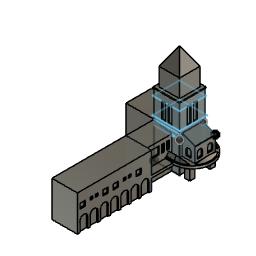
theater (Autodesk Fusion 360 design; units mm, degrees)
Autodesk Fusion 360 part; units mm, degrees
note: some values were not read from the file. Set by a fixed rule: which sketch regions a step uses.
sketch "Sketch1" plane through (0, 0, 0) normal (0, 0, 1) x (1, 0, 0)
  line L0 (-50, 50) -> (50, 50)
  line L1 (50, 50) -> (50, -50)
  line L2 (50, -50) -> (-50, -50)
  line L3 (-50, -50) -> (-50, 50)
  constraint horizontal L0
  constraint vertical L1
  constraint horizontal L2
  constraint vertical L3
extrude "Extrude1" add sketch "Sketch1" along normal blind 325
sketch "Sketch2" plane through (0, 0, 325) normal (0, 0, 1) x (-1, 0, 0)
  line L0 (50, 50) -> (-50, 50)
  line L1 (-50, 50) -> (-50, -50)
  line L2 (-50, -50) -> (50, -50)
  line L3 (50, -50) -> (50, 50)
  line L4 (40, -40) -> (-40, -40)
  line L5 (-40, -40) -> (-40, 40)
  line L6 (-40, 40) -> (40, 40)
  line L7 (40, 40) -> (40, -40)
  constraint horizontal L4
  constraint vertical L5
  constraint horizontal L6
  constraint vertical L7
extrude "Extrude2" cut sketch "Sketch2" against normal blind 50 contours L0 L1 L2 L3 | L4 L5 L6 L7
sketch "Sketch3" plane through (0, 0, 275) normal (0, 0, 1) x (-1, 0, 0)
  line L0 (50, -50) -> (50, 50)
  line L1 (50, 50) -> (-50, 50)
  line L2 (-50, 50) -> (-50, -50)
  line L3 (-50, -50) -> (50, -50)
  line L4 (40, -40) -> (-40, -40)
  line L5 (-40, -40) -> (-40, 40)
  line L6 (-40, 40) -> (40, 40)
  line L7 (40, 40) -> (40, -40)
  constraint horizontal L4
  constraint vertical L5
  constraint horizontal L6
  constraint vertical L7
extrude "Extrude3" add sketch "Sketch3" along normal blind 70 contours L4 L5 L6 L7
extrude "Extrude4" cut 1 faces at (-13.3333, 13.3333, 345) along direction (0, 0, -1) blind 25
extrude "Extrude5" cut 1 faces at (46.6667, 13.3333, 275) along direction (0, 0, -1) blind 25
extrude "Extrude6" add 1 faces at (-13.3333, 13.3333, 320) along direction (0, 0, 1) blind 80 draft -30
sketch "Sketch4" plane through (0, 0, 0) normal (0, 0, 1) x (1, 0, 0)
sketch "Sketch5" plane through (0, 0, 250) normal (0, 0, 1) x (-1, 0, 0)
  line L0 (40, 40) -> (40, -40)
  line L1 (40, -40) -> (-40, -40)
  line L2 (-40, -40) -> (-40, 40)
  line L3 (-40, 40) -> (40, 40)
  line L4 (50, -50) -> (50, 50)
  line L5 (50, 50) -> (-50, 50)
  line L6 (-50, 50) -> (-50, -50)
  line L7 (-50, -50) -> (50, -50)
  line L8 (52, -52) -> (-52, -52)
  line L9 (-52, -52) -> (-52, 52)
  line L10 (-52, 52) -> (52, 52)
  line L11 (52, 52) -> (52, -52)
  constraint horizontal L8
  constraint vertical L9
  constraint horizontal L10
  constraint vertical L11
extrude "Extrude7" add sketch "Sketch5" against normal blind 3.5 contours L8 L9 L10 L11
extrude "Extrude8" add 1 faces at (-16.6667, 51.3333, 246.5) along direction (0, 0, -1) blind 5 draft -60
sketch "Sketch6" plane through (50, 0, 0) normal (1, 0, 0) x (0, 1, 0)
  line L0 (50, 246.5) -> (-50, 246.5)
  line L1 (-50, 246.5) -> (-50, 0)
  line L2 (-50, 0) -> (50, 0)
  line L3 (50, 0) -> (50, 246.5)
  line L4 (-40, 120) -> (40, 120)
  line L5 (40, 120) -> (40, 60)
  line L6 (40, 60) -> (-40, 60)
  line L7 (-40, 60) -> (-40, 120)
  line L8 (-40, 100) -> (40, 100)
  line L9 (40, 100) -> (40, 60)
  line L10 (40, 60) -> (-40, 60)
  line L11 (-40, 60) -> (-40, 100)
  constraint horizontal L4
  constraint vertical L5
  constraint horizontal L6
  constraint vertical L7
  constraint horizontal L8
  constraint vertical L9
  constraint horizontal L10
  constraint vertical L11
  constraint coincident L7 L8.start
extrude "Extrude9" add sketch "Sketch6" along normal blind 50 contours L4 L5 L7 L8 | L5 L6 L7 L8 L9 L10 L11
sketch "Sketch7" plane through (100, 0, 0) normal (1, 0, 0) x (0, 1, 0)
  line L0 (-40, 60) -> (40, 60)
  line L1 (40, 60) -> (40, 120)
  line L2 (40, 120) -> (-40, 120)
  line L3 (-40, 120) -> (-40, 60)
  line L4 (-40, 120) -> (40, 120)
  line L5 (40, 120) -> (40, 100)
  line L6 (40, 100) -> (-40, 100)
  line L7 (-40, 100) -> (-40, 120)
  constraint horizontal L4
  constraint vertical L5
  constraint horizontal L6
  constraint vertical L7
  constraint coincident L1 L5.end
  constraint coincident L2.end L3.start
extrude "Extrude10" add sketch "Sketch7" against normal blind 50 draft 20 contours L1 L2 L3 L4 L5 L6 L7
sketch "Sketch8" plane through (50, 0, 0) normal (1, 0, 0) x (0, 1, 0)
  line L0 (-50, 138.1985) -> (50, 138.1985)
  line L1 (50, 138.1985) -> (50, 246.5)
  line L2 (50, 246.5) -> (-50, 246.5)
  line L3 (-50, 246.5) -> (-50, 138.1985)
  line L4 (-40, 60) -> (-60, 60)
  line L5 (-60, 60) -> (-60, 140)
  line L6 (-60, 140) -> (-40, 140)
  line L7 (-40, 140) -> (-40, 60)
  line L8 (60, 60) -> (40, 60)
  line L9 (40, 60) -> (40, 140)
  line L10 (40, 140) -> (60, 140)
  line L11 (60, 140) -> (60, 60)
  constraint horizontal L4
  constraint vertical L5
  constraint horizontal L6
  constraint vertical L7
  constraint horizontal L8
  constraint vertical L9
  constraint horizontal L10
  constraint vertical L11
extrude "Extrude11" cut sketch "Sketch8" along normal blind 140 contours L0 L1 L8 L9 L10 L11
sketch "Sketch9" plane through (50, 0, 0) normal (1, 0, 0) x (0, 1, 0)
  line L0 (-50, 138.1985) -> (40, 138.1985)
  line L1 (40, 138.1985) -> (40, 60)
  line L2 (40, 60) -> (-40, 60)
  line L3 (-40, 60) -> (-40, 81.8015)
  line L4 (-40, 81.8015) -> (-50, 81.8015)
  line L5 (-50, 81.8015) -> (-50, 0)
  line L6 (-50, 0) -> (50, 0)
  line L7 (50, 0) -> (50, 246.5)
  line L8 (50, 246.5) -> (-50, 246.5)
  line L9 (-50, 246.5) -> (-50, 138.1985)
  line L10 (-40, 60) -> (-61.5623, 60)
  line L11 (-61.5623, 60) -> (-61.5623, 138.1985)
  line L12 (-61.5623, 138.1985) -> (-40, 138.1985)
  line L13 (-40, 138.1985) -> (-40, 60)
  constraint horizontal L10
  constraint vertical L11
  constraint horizontal L12
  constraint vertical L13
  constraint coincident L2.end L3.start
extrude "Extrude12" cut sketch "Sketch9" along normal blind 320 contours L0 L4 L5 L10 L11 L12 L13
sketch "Sketch10" plane through (100, 0, 0) normal (1, 0, 0) x (0, 1, 0)
  line L0 (-40, 120) -> (-40, 60)
  line L1 (-40, 60) -> (40, 60)
  line L2 (40, 60) -> (40, 120)
  line L3 (40, 120) -> (-40, 120)
  line L4 (-30, 70) -> (-10, 70)
  line L5 (-10, 70) -> (-10, 90)
  line L6 (-10, 90) -> (-30, 90)
  line L7 (-30, 90) -> (-30, 70)
  circle A0 centre (-20, 90) radius 10
  line L8 (-30, 90) -> (-10, 90)
  line L9 (-30, 90) -> (-10, 90)
  constraint horizontal L4
  constraint vertical L5
  constraint horizontal L6
  constraint vertical L7
  constraint midpoint L6 A0.centre
  constraint coincident L5.end A0
extrude "Extrude13" cut sketch "Sketch10" against normal blind 5 contours L4 L5 L7 A0 | L6 A0 L8 L9 | L6 A0 L8 L9
sketch "Sketch11" plane through (100, 0, 0) normal (1, 0, 0) x (0, 1, 0)
  line L0 (-30, 70) -> (-30, 90)
  arc A0 (-10, 90) -> (-30, 90) centre (-20, 90) ccw
  line L1 (-10, 90) -> (-10, 70)
  line L2 (-10, 70) -> (-30, 70)
  line L3 (-40, 120) -> (-40, 60)
  line L4 (-40, 60) -> (40, 60)
  line L5 (40, 60) -> (40, 120)
  line L6 (40, 120) -> (-40, 120)
  line L7 (10, 70) -> (30, 70)
  line L8 (30, 70) -> (30, 90)
  line L9 (30, 90) -> (10, 90)
  line L10 (10, 90) -> (10, 70)
  circle A1 centre (20, 90) radius 10
  constraint horizontal L7
  constraint vertical L8
  constraint horizontal L9
  constraint vertical L10
  constraint midpoint L9 A1.centre
  constraint coincident L8.end A1
extrude "Extrude14" cut sketch "Sketch11" against normal blind 5 contours L7 L8 L10 A1 | L9 A1 | L9 A1
sketch "Sketch12" plane through (0, 40, 0) normal (0, 1, 0) x (-1, 0, 0)
  line L0 (-100, 120) -> (-100, 60)
  line L1 (-100, 60) -> (-50, 60)
  line L2 (-50, 60) -> (-50, 138.1985)
  line L3 (-50, 138.1985) -> (-100, 120)
  line L4 (-85, 70) -> (-65, 70)
  line L5 (-65, 70) -> (-65, 90)
  line L6 (-65, 90) -> (-85, 90)
  line L7 (-85, 90) -> (-85, 70)
  circle A0 centre (-75, 90) radius 10
  constraint horizontal L4
  constraint vertical L5
  constraint horizontal L6
  constraint vertical L7
  constraint midpoint L6 A0.centre
  constraint coincident L5.end A0
extrude "Extrude15" cut sketch "Sketch12" against normal blind 5 contours L4 L5 L7 A0 | L6 A0 | L6 A0
sketch "Sketch13" plane through (0, -40, 0) normal (0, -1, 0) x (1, 0, 0)
  line L0 (50, 138.1985) -> (50, 60)
  line L1 (50, 60) -> (100, 60)
  line L2 (100, 60) -> (100, 120)
  line L3 (100, 120) -> (50, 138.1985)
sketch "Sketch14" plane through (0, -40, 0) normal (0, -1, 0) x (1, 0, 0)
  line L0 (65, 70) -> (85, 70)
  line L1 (85, 70) -> (85, 90)
  line L2 (85, 90) -> (65, 90)
  line L3 (65, 90) -> (65, 70)
  circle A0 centre (75, 90) radius 10
  constraint horizontal L0
  constraint vertical L1
  constraint horizontal L2
  constraint vertical L3
  constraint midpoint L2 A0.centre
  constraint coincident L1.end A0
extrude "Extrude16" cut sketch "Sketch14" against normal blind 5
sketch "Sketch15" plane through (50.265, 0, 138.102) normal (0.34202, 0, 0.939693) x (0, 1, 0)
  line L0 (-40, 0.282) -> (-40, -52.9268)
  line L1 (-40, -52.9268) -> (40, -52.9268)
  line L2 (40, -52.9268) -> (40, 0.282)
  line L3 (40, 0.282) -> (-40, 0.282)
sketch "Sketch16" plane through (100, 0, 0) normal (1, 0, 0) x (0, 1, 0)
  line L0 (10, 70) -> (10, 90)
  arc A0 (30, 90) -> (10, 90) centre (20, 90) ccw
  line L1 (30, 90) -> (30, 70)
  line L2 (30, 70) -> (10, 70)
  line L3 (-30, 70) -> (-30, 90)
  arc A1 (-10, 90) -> (-30, 90) centre (-20, 90) ccw
  line L4 (-10, 90) -> (-10, 70)
  line L5 (-10, 70) -> (-30, 70)
  line L6 (-40, 120) -> (-40, 60)
  line L7 (-40, 60) -> (40, 60)
  line L8 (40, 60) -> (40, 120)
  line L9 (40, 120) -> (-40, 120)
  line L10 (-40, 120) -> (40, 120)
  line L11 (40, 120) -> (40, 117.9644)
  line L12 (40, 117.9644) -> (-40, 117.9644)
  line L13 (-40, 117.9644) -> (-40, 120)
  constraint horizontal L10
  constraint vertical L11
  constraint horizontal L12
  constraint vertical L13
  constraint coincident L8 L11.end
  constraint coincident L6.start L9.end
extrude "Extrude17" add sketch "Sketch16" along normal blind 4 draft -20 contours L6 L8 L9 L10 L11 L12 L13
sketch "Sketch17" plane through (0, 40, 0) normal (0, 1, 0) x (-1, 0, 0)
  line L0 (-85, 70) -> (-85, 90)
  arc A0 (-65, 90) -> (-85, 90) centre (-75, 90) ccw
  line L1 (-65, 90) -> (-65, 70)
  line L2 (-65, 70) -> (-85, 70)
  line L3 (-100, 117.9644) -> (-100, 60)
  line L4 (-100, 60) -> (-50, 60)
  line L5 (-50, 60) -> (-50, 138.1985)
  line L6 (-50, 138.1985) -> (-100, 120)
  line L7 (-100, 120) -> (-100, 117.9644)
  line L8 (-100, 117.9644) -> (-50, 136.0984)
  constraint coincident L3.start L7.end
  constraint coincident L5 L8.end
ref_plane "WorkPlane1" through (0, 0, 60) normal (0, 0, 1) x (1, 0, 0)
sketch "Sketch18" plane through (0, 0, 60) normal (0, 0, 1) x (1, 0, 0)
  circle A0 centre (50, 0) radius 76.0694
extrude "Extrude18" add sketch "Sketch18" against normal blind 10
sketch "Sketch19" plane through (0, 0, 60) normal (0, 0, 1) x (-1, 0, 0)
  line L0 (-50, 50) -> (7.3284, 50)
  arc A0 (7.3284, 50) -> (7.3284, -50) centre (-50, 0) ccw
  line L1 (7.3284, -50) -> (-50, -50)
  line L2 (-50, -50) -> (-50, -40)
  line L3 (-50, -40) -> (-100, -40)
  line L4 (-100, -40) -> (-100, 40)
  line L5 (-100, 40) -> (-50, 40)
  line L6 (-50, 40) -> (-50, 50)
  line L7 (-104.9015, -44.9015) -> (-104.9015, 44.9015)
  line L8 (-54.9015, 54.9015) -> (-4.7156, 54.9015)
  arc A1 (-4.7156, 54.9015) -> (-4.7156, -54.9015) centre (-50, 0) ccw
  line L9 (-4.7156, -54.9015) -> (-54.9015, -54.9015)
  line L10 (-54.9015, 54.9015) -> (-95.2844, 54.9015)
  line L11 (-54.9015, -54.9015) -> (-95.2844, -54.9015)
  line L12 (-104.9015, 49.6433) -> (-104.9015, -50)
  constraint coincident A1 L10.end
  constraint concentric A0 A1
  constraint coincident A1 L11.end
  constraint parallel L7 L12
extrude "Extrude19" add sketch "Sketch19" along normal blind 20 draft -30 contours L7 A1 L12 | L8 A1 L10 | A1 L9 L11
sketch "Sketch20" plane through (0, 0, 50) normal (0, 0, -1) x (1, 0, 0)
  line L0 (-7.3284, 50) -> (50, 50)
  line L1 (50, 50) -> (50, -50)
  line L2 (50, -50) -> (-7.3284, -50)
  arc A0 (-7.3284, -50) -> (-7.3284, 50) centre (50, 0) ccw
  line L3 (90, 50) -> (70, 50)
  line L4 (70, 50) -> (70, 30)
  line L5 (70, 30) -> (90, 30)
  line L6 (90, 30) -> (90, 50)
  line L7 (70, -50) -> (90, -50)
  line L8 (90, -50) -> (90, -30)
  line L9 (90, -30) -> (70, -30)
  line L10 (70, -30) -> (70, -50)
  constraint horizontal L3
  constraint vertical L4
  constraint horizontal L5
  constraint vertical L6
  constraint horizontal L7
  constraint vertical L8
  constraint horizontal L9
  constraint vertical L10
extrude "Extrude20" add sketch "Sketch20" along normal blind 50 contours L3 L4 L5 L6 | L7 L8 L9 L10
sketch "Sketch21" plane through (0, -50, 0) normal (0, -1, 0) x (1, 0, 0)
  line L0 (-7.3284, 60) -> (50, 60)
  line L1 (50, 60) -> (50, 246.5)
  line L2 (50, 246.5) -> (-50, 246.5)
  line L3 (-50, 246.5) -> (-50, 0)
  line L4 (-50, 0) -> (50, 0)
  line L5 (50, 0) -> (50, 50)
  line L6 (50, 50) -> (-7.3284, 50)
  line L7 (-7.3284, 50) -> (-7.3284, 60)
  line L8 (50, 120) -> (-50, 120)
  line L9 (-50, 120) -> (-50, 0)
  line L10 (-50, 0) -> (50, 0)
  line L11 (50, 0) -> (50, 120)
  constraint horizontal L8
  constraint vertical L9
  constraint horizontal L10
  constraint vertical L11
  constraint coincident L3.end L4.start
  constraint coincident L1 L8.start
sketch "Sketch22" plane through (0, -50, 60) normal (0, -1, 0) x (1, 0, 0)
sketch "Sketch23" plane through (0, 0, 0) normal (0, 0, 1) x (1, 0, 0)
  line L0 (-50, -50) -> (50, -50)
  line L1 (50, -50) -> (50, -90)
  line L2 (50, -90) -> (-50, -90)
  line L3 (-50, -90) -> (-50, -50)
  line L4 (50, 50) -> (-50, 50)
  line L5 (-50, 50) -> (-50, 90)
  line L6 (-50, 90) -> (50, 90)
  line L7 (50, 90) -> (50, 50)
  constraint horizontal L0
  constraint vertical L1
  constraint horizontal L2
  constraint vertical L3
  constraint horizontal L4
  constraint vertical L5
  constraint horizontal L6
  constraint vertical L7
extrude "Extrude21" add sketch "Sketch23" along normal blind 120 contours L0 L1 L2 L3
sketch "Sketch24" plane through (0, -50, 183.25) normal (0, -1, 0) x (1, 0, 0)
extrude "Extrude22" add 1 faces at (16.6667, -90, 80) along direction (0, -1, 0) blind 70
ref_plane "WorkPlane2" through (50, 0, 0) normal (1, 0, 0) x (0, 1, 0)
sketch "Sketch25" plane through (50, 0, 0) normal (1, 0, 0) x (0, 1, 0)
  line L0 (-160, 120) -> (-50, 120)
  line L1 (-50, 120) -> (-50, 138)
  line L2 (-50, 138) -> (-160, 138)
  line L3 (-160, 138) -> (-160, 120)
  constraint horizontal L0
  constraint vertical L1
  constraint horizontal L2
  constraint vertical L3
extrude "Extrude23" add 1 faces at (-16.6667, -123.3333, 120) along direction (0, 0, 1) blind 20
sketch "Sketch26" plane through (0, -160, 0) normal (0, -1, 0) x (1, 0, 0)
  line L0 (-50, 0) -> (50, 0)
  line L1 (50, 0) -> (50, 140)
  line L2 (50, 140) -> (-50, 140)
  line L3 (-50, 140) -> (-50, 0)
sketch "Sketch27" plane through (0, -50, 0) normal (0, -1, 0) x (1, 0, 0)
  line L0 (50, 120) -> (-50, 140)
  line L1 (-50, 140) -> (50, 140)
  line L2 (50, 140) -> (50, 120)
  constraint horizontal L1
  constraint perpendicular L1 L2
sketch "Sketch28" plane through (0, -160, 70) normal (0, -1, 0) x (1, 0, 0)
  line L0 (50, 50) -> (50, 70)
  line L1 (50, 70) -> (-50, 70)
  line L2 (-50, 70) -> (50, 50)
  constraint vertical L0
  constraint perpendicular L0 L1
extrude "Extrude24" cut sketch "Sketch28" against normal blind 110
sketch "Sketch29" plane through (0, -50, 0) normal (0, -1, 0) x (1, 0, 0)
sketch "Sketch30" plane through (0, 0, 0) normal (0, 0, 1) x (1, 0, 0)
  line L0 (-50, -160) -> (50, -160)
  line L1 (50, -160) -> (50, -450.3977)
  line L2 (50, -450.3977) -> (-50, -450.3977)
  line L3 (-50, -450.3977) -> (-50, -160)
  constraint horizontal L0
  constraint vertical L1
  constraint horizontal L2
  constraint vertical L3
sketch "Sketch31" plane through (0, 0, 0) normal (0, 0, 1) x (1, 0, 0)
extrude "Extrude25" add sketch "Sketch30" along normal blind 140
sketch "Sketch32" plane through (0, -160, 0) normal (0, -1, 0) x (1, 0, 0)
sketch "Sketch33" plane through (50, 0, 0) normal (1, 0, 0) x (0, 1, 0)
  line L0 (-50, 120) -> (-160, 120)
  line L1 (-160, 120) -> (-160, 140)
  line L2 (-160, 140) -> (-450.3977, 140)
  line L3 (-450.3977, 140) -> (-450.3977, 0)
  line L4 (-450.3977, 0) -> (50, 0)
  line L5 (50, 0) -> (50, 50)
  line L6 (50, 50) -> (-76.0694, 50)
  line L7 (-76.0694, 50) -> (-76.0694, 60)
  line L8 (-76.0694, 60) -> (-71.1678, 60)
  line L9 (-71.1678, 60) -> (-63.0347, 74.087)
  line L10 (-63.0347, 74.087) -> (-54.9015, 60)
  line L11 (-54.9015, 60) -> (-40, 60)
  line L12 (-40, 60) -> (-40, 138.1985)
  line L13 (-40, 138.1985) -> (40, 138.1985)
  line L14 (40, 138.1985) -> (40, 60)
  line L15 (40, 60) -> (50, 60)
  line L16 (50, 60) -> (50, 246.5)
  line L17 (50, 246.5) -> (-50, 246.5)
  line L18 (-50, 246.5) -> (-50, 120)
  line L19 (-160, 120) -> (-50, 120)
  line L20 (-50, 120) -> (-50, 0)
  line L21 (-50, 0) -> (-160, 0)
  line L22 (-160, 0) -> (-160, 120)
  constraint horizontal L19
  constraint vertical L20
  constraint horizontal L21
  constraint vertical L22
  constraint coincident L4 L20.end
  constraint coincident L0.end L1.start
extrude "Extrude26" cut sketch "Sketch33" against normal blind 30 contours L0 L4 L6 L7 L8 L9 L10 L11 L19 L20 L21 L22
extrude "Extrude27" cut sketch "Sketch25" against normal blind 30
sketch "Sketch34" plane through (0, -160, 70) normal (0, -1, 0) x (1, 0, 0)
  line L0 (20, -15) -> (50, -15)
  line L1 (50, -15) -> (50, -25)
  line L2 (50, -25) -> (20, -25)
  line L3 (20, -25) -> (20, -15)
  constraint horizontal L0
  constraint vertical L1
  constraint horizontal L2
  constraint vertical L3
extrude "Extrude28" add sketch "Sketch34" against normal blind 110
sketch "Sketch35" plane through (50, 0, 0) normal (1, 0, 0) x (0, 1, 0)
  line L0 (-160, 0) -> (-160, 45)
  line L1 (-160, 45) -> (-50, 45)
  line L2 (-50, 45) -> (-50, 0)
  line L3 (-50, 0) -> (50, 0)
  line L4 (50, 0) -> (50, 50)
  line L5 (50, 50) -> (-76.0694, 50)
  line L6 (-76.0694, 50) -> (-76.0694, 55)
  line L7 (-76.0694, 55) -> (-160, 55)
  line L8 (-160, 55) -> (-160, 140)
  line L9 (-160, 140) -> (-450.3977, 140)
  line L10 (-450.3977, 140) -> (-450.3977, 0)
  line L11 (-450.3977, 0) -> (-160, 0)
  line L12 (-440, 0) -> (-410, 0)
  line L13 (-410, 0) -> (-410, 40)
  line L14 (-410, 40) -> (-440, 40)
  line L15 (-440, 40) -> (-440, 0)
  line L16 (-400, 0) -> (-370, 0)
  line L17 (-370, 0) -> (-370, 40)
  line L18 (-370, 40) -> (-400, 40)
  line L19 (-400, 40) -> (-400, 0)
  line L20 (-360, 0) -> (-330, 0)
  line L21 (-330, 0) -> (-330, 40)
  line L22 (-330, 40) -> (-360, 40)
  line L23 (-360, 40) -> (-360, 0)
  line L24 (-320, 0) -> (-290, 0)
  line L25 (-290, 0) -> (-290, 40)
  line L26 (-290, 40) -> (-320, 40)
  line L27 (-320, 40) -> (-320, 0)
  line L28 (-280, 0) -> (-250, 0)
  line L29 (-250, 0) -> (-250, 40)
  line L30 (-250, 40) -> (-280, 40)
  line L31 (-280, 40) -> (-280, 0)
  line L32 (-240, 0) -> (-210, 0)
  line L33 (-210, 0) -> (-210, 40)
  line L34 (-210, 40) -> (-240, 40)
  line L35 (-240, 40) -> (-240, 0)
  line L36 (-200, 0) -> (-170, 0)
  line L37 (-170, 0) -> (-170, 40)
  line L38 (-170, 40) -> (-200, 40)
  line L39 (-200, 40) -> (-200, 0)
  circle A0 centre (-425, 40) radius 15.3222
  circle A1 centre (-385, 40) radius 15
  circle A2 centre (-345, 40) radius 15.4824
  circle A3 centre (-305, 40) radius 15
  circle A4 centre (-265, 40) radius 15.574
  circle A5 centre (-225, 40) radius 15
  circle A6 centre (-185, 40) radius 15
  line L40 (-440, 100) -> (-420, 100)
  line L41 (-420, 100) -> (-420, 80)
  line L42 (-420, 80) -> (-440, 80)
  line L43 (-440, 80) -> (-440, 100)
  line L44 (-400, 100) -> (-390, 100)
  line L45 (-390, 100) -> (-390, 90)
  line L46 (-390, 90) -> (-400, 90)
  line L47 (-400, 90) -> (-400, 100)
  line L48 (-380, 100) -> (-370, 100)
  line L49 (-370, 100) -> (-370, 90)
  line L50 (-370, 90) -> (-380, 90)
  line L51 (-380, 90) -> (-380, 100)
  line L52 (-350, 100) -> (-330, 100)
  line L53 (-330, 100) -> (-330, 80)
  line L54 (-330, 80) -> (-350, 80)
  line L55 (-350, 80) -> (-350, 100)
  line L56 (-310, 100) -> (-290, 100)
  line L57 (-290, 100) -> (-290, 80)
  line L58 (-290, 80) -> (-310, 80)
  line L59 (-310, 80) -> (-310, 100)
  line L60 (-270, 100) -> (-260, 100)
  line L61 (-260, 100) -> (-260, 90)
  line L62 (-260, 90) -> (-270, 90)
  line L63 (-270, 90) -> (-270, 100)
  line L64 (-250, 100) -> (-240, 100)
  line L65 (-240, 100) -> (-240, 90)
  line L66 (-240, 90) -> (-250, 90)
  line L67 (-250, 90) -> (-250, 100)
  line L68 (-220, 100) -> (-200, 100)
  line L69 (-200, 100) -> (-200, 80)
  line L70 (-200, 80) -> (-220, 80)
  line L71 (-220, 80) -> (-220, 100)
  constraint horizontal L12
  constraint vertical L13
  constraint horizontal L14
  constraint vertical L15
  constraint coincident L11 L12.start
  constraint horizontal L16
  constraint vertical L17
  constraint horizontal L18
  constraint vertical L19
  constraint coincident L11 L16.start
  constraint horizontal L20
  constraint vertical L21
  constraint horizontal L22
  constraint vertical L23
  constraint coincident L11 L20.start
  constraint horizontal L24
  constraint vertical L25
  constraint horizontal L26
  constraint vertical L27
  constraint coincident L11 L24.start
  constraint horizontal L28
  constraint vertical L29
  constraint horizontal L30
  constraint vertical L31
  constraint coincident L11 L28.start
  constraint horizontal L32
  constraint vertical L33
  constraint horizontal L34
  constraint vertical L35
  constraint coincident L11 L32.start
  constraint horizontal L36
  constraint vertical L37
  constraint horizontal L38
  constraint vertical L39
  constraint coincident L11 L36.start
  constraint midpoint L14 A0.centre
  constraint midpoint L18 A1.centre
  constraint coincident L17.end A1
  constraint midpoint L22 A2.centre
  constraint midpoint L26 A3.centre
  constraint coincident L25.end A3
  constraint midpoint L30 A4.centre
  constraint midpoint L34 A5.centre
  constraint coincident L33.end A5
  constraint midpoint L38 A6.centre
  constraint coincident L37.end A6
  constraint horizontal L40
  constraint vertical L41
  constraint horizontal L42
  constraint vertical L43
  constraint horizontal L44
  constraint vertical L45
  constraint horizontal L46
  constraint vertical L47
  constraint horizontal L48
  constraint vertical L49
  constraint horizontal L50
  constraint vertical L51
  constraint horizontal L52
  constraint vertical L53
  constraint horizontal L54
  constraint vertical L55
  constraint horizontal L56
  constraint vertical L57
  constraint horizontal L58
  constraint vertical L59
  constraint horizontal L60
  constraint vertical L61
  constraint horizontal L62
  constraint vertical L63
  constraint horizontal L64
  constraint vertical L65
  constraint horizontal L66
  constraint vertical L67
  constraint horizontal L68
  constraint vertical L69
  constraint horizontal L70
  constraint vertical L71
extrude "Extrude29" cut sketch "Sketch35" against normal blind 5 contours L11 L36 L37 L39 A6 | L38 A6 | L38 A6 | L11 L32 L33 L35 A5 | L34 A5 | L34 A5 | L11 L28 L29 L31 A4 | L29 L30 L31 A4 | L29 L30 L31 A4 | L11 L24 L25 L27 A3 | L26 A3 | L26 A3 | L11 L20 L21 L23 A2 | L21 L22 L23 A2 | L21 L22 L23 A2 | L11 L16 L17 L19 A1 | L11 L12 L13 L15 A0 | L18 A1 | L18 A1 | L13 L14 L15 A0 | L13 L14 L15 A0 | L40 L41 L42 L43 | L44 L45 L46 L47 | L48 L49 L50 L51 | L52 L53 L54 L55 | L56 L57 L58 L59 | L60 L61 L62 L63 | L64 L65 L66 L67 | L68 L69 L70 L71
sketch "Sketch36" plane through (20, 0, 0) normal (1, 0, 0) x (0, 1, 0)
  line L0 (-160, 55) -> (-76.0694, 55)
  line L1 (-76.0694, 55) -> (-76.0694, 60)
  line L2 (-76.0694, 60) -> (-71.1678, 60)
  line L3 (-71.1678, 60) -> (-63.0347, 74.087)
  line L4 (-63.0347, 74.087) -> (-54.9015, 60)
  line L5 (-54.9015, 60) -> (-50, 60)
  line L6 (-50, 60) -> (-50, 126)
  line L7 (-50, 126) -> (-160, 126)
  line L8 (-160, 126) -> (-160, 55)
  line L9 (-150, 110) -> (-140, 110)
  line L10 (-140, 110) -> (-140, 80)
  line L11 (-140, 80) -> (-150, 80)
  line L12 (-150, 80) -> (-150, 110)
  line L13 (-130, 110) -> (-100, 110)
  line L14 (-100, 110) -> (-100, 80)
  line L15 (-100, 80) -> (-130, 80)
  line L16 (-130, 80) -> (-130, 110)
  line L17 (-90, 110) -> (-80, 110)
  line L18 (-80, 110) -> (-80, 80)
  line L19 (-80, 80) -> (-90, 80)
  line L20 (-90, 80) -> (-90, 110)
  line L21 (-70, 110) -> (-60, 110)
  line L22 (-60, 110) -> (-60, 80)
  line L23 (-60, 80) -> (-70, 80)
  line L24 (-70, 80) -> (-70, 110)
  constraint horizontal L9
  constraint vertical L10
  constraint horizontal L11
  constraint vertical L12
  constraint horizontal L13
  constraint vertical L14
  constraint horizontal L15
  constraint vertical L16
  constraint horizontal L17
  constraint vertical L18
  constraint horizontal L19
  constraint vertical L20
  constraint horizontal L21
  constraint vertical L22
  constraint horizontal L23
  constraint vertical L24
extrude "Extrude30" cut sketch "Sketch36" against normal blind 5 contours L9 L10 L11 L12 | L13 L14 L15 L16 | L17 L18 L19 L20 | L21 L22 L23 L24
sketch "Sketch37" plane through (50, 0, 0) normal (1, 0, 0) x (0, 1, 0)
  line L0 (-50, 246.5) -> (-50, 60)
  line L1 (-50, 60) -> (-40, 60)
  line L2 (-40, 60) -> (-40, 138.1985)
  line L3 (-40, 138.1985) -> (40, 138.1985)
  line L4 (40, 138.1985) -> (40, 60)
  line L5 (40, 60) -> (50, 60)
  line L6 (50, 60) -> (50, 246.5)
  line L7 (50, 246.5) -> (-50, 246.5)
sketch "Sketch38" plane through (50, 0, 153.25) normal (1, 0, 0) x (0, 1, 0)
  line L0 (-5, 65) -> (-20, 65)
  line L1 (-20, 65) -> (-20, 0)
  line L2 (-20, 0) -> (-5, 0)
  line L3 (-5, 0) -> (-5, 65)
  line L4 (5, 0) -> (20, 0)
  line L5 (20, 0) -> (20, 65)
  line L6 (20, 65) -> (5, 65)
  line L7 (5, 65) -> (5, 0)
  constraint horizontal L0
  constraint vertical L1
  constraint horizontal L2
  constraint vertical L3
  constraint horizontal L4
  constraint vertical L5
  constraint horizontal L6
  constraint vertical L7
sketch "Sketch39" plane through (0, 50, 0) normal (0, 1, 0) x (-1, 0, 0)
  line L0 (-50, 60) -> (7.3284, 60)
  line L1 (7.3284, 60) -> (7.3284, 50)
  line L2 (7.3284, 50) -> (-50, 50)
  line L3 (-50, 50) -> (-50, 0)
  line L4 (-50, 0) -> (50, 0)
  line L5 (50, 0) -> (50, 246.5)
  line L6 (50, 246.5) -> (-50, 246.5)
  line L7 (-50, 246.5) -> (-50, 60)
ref_plane "WorkPlane3" through (50, 5, 153.25) normal (0, 0, -1) x (-1, 0, 0)
sketch "Sketch40" plane through (50, 5, 153.25) normal (0, 0, -1) x (-1, 0, 0)
  line L0 (-3.3107, -57.3854) -> (103.3673, -57.3854)
  line L1 (103.3673, -57.3854) -> (103.3673, 49.2926)
  line L2 (103.3673, 49.2926) -> (-3.3107, 49.2926)
  line L3 (-3.3107, 49.2926) -> (-3.3107, -57.3854)
  constraint horizontal L0
  constraint vertical L1
  constraint horizontal L2
  constraint vertical L3
ref_plane "WorkPlane4" through (50, 20, 218.25) normal (0, 0, 1) x (1, 0, 0)
sketch "Sketch41" plane through (50, 20, 218.25) normal (0, 0, 1) x (1, 0, 0)
  line L0 (0, -70) -> (-104.103, -70)
  line L1 (-104.103, -70) -> (-104.103, 33.1069)
  line L2 (-104.103, 33.1069) -> (0, 33.1069)
  line L3 (0, 33.1069) -> (0, -70)
  constraint horizontal L0
  constraint vertical L1
  constraint horizontal L2
  constraint vertical L3
sketch "Sketch42" plane through (0, 50, 123.25) normal (0, 1, 0) x (-1, 0, 0)
  line L0 (-5, 95) -> (-20, 95)
  line L1 (-20, 95) -> (-20, 30)
  line L2 (-20, 30) -> (-5, 30)
  line L3 (-5, 30) -> (-5, 95)
  line L4 (5, 95) -> (20, 95)
  line L5 (20, 95) -> (20, 30)
  line L6 (20, 30) -> (5, 30)
  line L7 (5, 30) -> (5, 95)
  constraint horizontal L0
  constraint vertical L1
  constraint horizontal L2
  constraint vertical L3
  constraint horizontal L4
  constraint vertical L5
  constraint horizontal L6
  constraint vertical L7
sketch "Sketch43" plane through (-50, 0, 0) normal (-1, 0, 0) x (0, -1, 0)
  line L0 (50, 246.5) -> (-50, 246.5)
  line L1 (-50, 246.5) -> (-50, 0)
  line L2 (-50, 0) -> (450.3977, 0)
  line L3 (450.3977, 0) -> (450.3977, 140)
  line L4 (450.3977, 140) -> (160, 140)
  line L5 (160, 140) -> (50, 140)
  line L6 (50, 140) -> (50, 246.5)
  line L7 (-19.8799, 152.8429) -> (-4.8735, 152.8429)
  line L8 (-4.8735, 152.8429) -> (-4.8735, 218.2707)
  line L9 (-4.8735, 218.2707) -> (-19.8799, 218.2707)
  line L10 (-19.8799, 218.2707) -> (-19.8799, 152.8429)
  line L11 (4.9706, 218.2707) -> (20.2171, 218.2707)
  line L12 (20.2171, 218.2707) -> (20.2171, 152.8429)
  line L13 (20.2171, 152.8429) -> (4.9706, 152.8429)
  line L14 (4.9706, 152.8429) -> (4.9706, 218.2707)
  constraint horizontal L7
  constraint vertical L8
  constraint horizontal L9
  constraint vertical L10
  constraint horizontal L11
  constraint vertical L12
  constraint horizontal L13
  constraint vertical L14
sketch "Sketch44" plane through (0, -50, 183.25) normal (0, -1, 0) x (1, 0, 0)
  line L0 (-20, 35) -> (-5, 35)
  line L1 (-5, 35) -> (-5, -30)
  line L2 (-5, -30) -> (-20, -30)
  line L3 (-20, -30) -> (-20, 35)
  line L4 (5, -30) -> (20, -30)
  line L5 (20, -30) -> (20, 35)
  line L6 (20, 35) -> (5, 35)
  line L7 (5, 35) -> (5, -30)
  constraint horizontal L0
  constraint vertical L1
  constraint horizontal L2
  constraint vertical L3
  constraint horizontal L4
  constraint vertical L5
  constraint horizontal L6
  constraint vertical L7
extrude "Extrude31" cut sketch "Sketch38" against normal blind 5
extrude "Extrude32" cut sketch "Sketch42" against normal blind 5
extrude "Extrude33" cut sketch "Sketch43" against normal blind 5 contours L7 L8 L9 L10 | L11 L12 L13 L14
extrude "Extrude34" cut sketch "Sketch44" against normal blind 5
sketch "Sketch45" plane through (-50, 0, 0) normal (-1, 0, 0) x (0, -1, 0)
  line L0 (-4.8735, 152.8429) -> (-19.8799, 152.8429)
  line L1 (-19.8799, 152.8429) -> (-19.8799, 218.2707)
  line L2 (-19.8799, 218.2707) -> (-4.8735, 218.2707)
  line L3 (-4.8735, 218.2707) -> (-4.8735, 152.8429)
  line L4 (20.2171, 218.2707) -> (20.2171, 152.8429)
  line L5 (20.2171, 152.8429) -> (4.9706, 152.8429)
  line L6 (4.9706, 152.8429) -> (4.9706, 218.2707)
  line L7 (4.9706, 218.2707) -> (20.2171, 218.2707)
  line L8 (50, 246.5) -> (-50, 246.5)
  line L9 (-50, 246.5) -> (-50, 0)
  line L10 (-50, 0) -> (450.3977, 0)
  line L11 (450.3977, 0) -> (450.3977, 140)
  line L12 (450.3977, 140) -> (160, 140)
  line L13 (160, 140) -> (50, 140)
  line L14 (50, 140) -> (50, 246.5)
  line L15 (50, 140) -> (-50, 140)
  line L16 (-50, 140) -> (-50, 0)
  line L17 (-50, 0) -> (50, 0)
  line L18 (50, 0) -> (50, 140)
  constraint horizontal L15
  constraint vertical L16
  constraint horizontal L17
  constraint vertical L18
  constraint coincident L9.end L10.start
  constraint coincident L13.end L14.start
extrude "Extrude35" add sketch "Sketch45" along normal blind 110 contours L9 L10 L15 L16 L17 L18
sketch "Sketch46" plane through (0, 50, 123.25) normal (0, 1, 0) x (-1, 0, 0)
  line L0 (-30, -10) -> (30, -10)
  line L1 (30, -10) -> (30, -60)
  line L2 (30, -60) -> (-30, -60)
  line L3 (-30, -60) -> (-30, -10)
  line L4 (70, 10) -> (90, 10)
  line L5 (90, 10) -> (90, -10)
  line L6 (90, -10) -> (70, -10)
  line L7 (70, -10) -> (70, 10)
  line L8 (101.642, 16.75) -> (121.642, 16.75)
  line L9 (121.642, 16.75) -> (121.642, 35)
  line L10 (121.642, 35) -> (101.642, 35)
  line L11 (101.642, 35) -> (101.642, 16.75)
  line L12 (50, -20) -> (160.1999, -20)
  line L13 (160.1999, -20) -> (160.1999, -123.6332)
  line L14 (160.1999, -123.6332) -> (50, -123.6332)
  line L15 (50, -123.6332) -> (50, -20)
  line L16 (121.6605, 16.75) -> (321.6087, 16.75)
  line L17 (321.6087, 16.75) -> (321.6087, -20)
  line L18 (321.6087, -20) -> (121.6605, -20)
  line L19 (121.6605, -20) -> (121.6605, 16.75)
  line L20 (321.6087, -20) -> (160.1999, -20)
  line L21 (160.1999, -20) -> (160.1999, -123.6332)
  line L22 (160.1999, -123.6332) -> (321.6087, -123.6332)
  line L23 (321.6087, -123.6332) -> (321.6087, -20)
  constraint horizontal L0
  constraint vertical L1
  constraint horizontal L2
  constraint vertical L3
  constraint horizontal L4
  constraint vertical L5
  constraint horizontal L6
  constraint vertical L7
  constraint horizontal L8
  constraint vertical L9
  constraint horizontal L10
  constraint vertical L11
  constraint horizontal L12
  constraint vertical L13
  constraint horizontal L14
  constraint vertical L15
  constraint horizontal L16
  constraint vertical L17
  constraint horizontal L18
  constraint vertical L19
  constraint horizontal L20
  constraint vertical L21
  constraint horizontal L22
  constraint vertical L23
extrude "Extrude36" add sketch "Sketch46" along normal blind 5 contours L0 L1 L2 L3
sketch "Sketch47" plane through (0, 55, 0) normal (0, 1, 0) x (-1, 0, 0)
  line L0 (-30, 63.25) -> (30, 63.25)
  line L1 (30, 63.25) -> (30, 113.25)
  line L2 (30, 113.25) -> (-30, 113.25)
  line L3 (-30, 113.25) -> (-30, 63.25)
  line L4 (-20, 100) -> (20, 100)
  line L5 (20, 100) -> (20, 70)
  line L6 (20, 70) -> (-20, 70)
  line L7 (-20, 70) -> (-20, 100)
  constraint horizontal L4
  constraint vertical L5
  constraint horizontal L6
  constraint vertical L7
extrude "Extrude37" cut sketch "Sketch47" against normal blind 5 contours L4 L5 L6 L7
sketch "Sketch48" plane through (0, 50, 0) normal (0, 1, 0) x (-1, 0, 0)
  line L0 (-30, 63.25) -> (-30, 113.25)
  line L1 (-30, 113.25) -> (30, 113.25)
  line L2 (30, 113.25) -> (30, 63.25)
  line L3 (30, 63.25) -> (-30, 63.25)
  line L4 (20, 218.25) -> (20, 153.25)
  line L5 (20, 153.25) -> (5, 153.25)
  line L6 (5, 153.25) -> (5, 218.25)
  line L7 (5, 218.25) -> (20, 218.25)
  line L8 (-20, 218.25) -> (-5, 218.25)
  line L9 (-5, 218.25) -> (-5, 153.25)
  line L10 (-5, 153.25) -> (-20, 153.25)
  line L11 (-20, 153.25) -> (-20, 218.25)
  line L12 (-50, 60) -> (7.3284, 60)
  line L13 (7.3284, 60) -> (7.3284, 50)
  line L14 (7.3284, 50) -> (-50, 50)
  line L15 (-50, 50) -> (-50, 0)
  line L16 (-50, 0) -> (160, 0)
  line L17 (160, 0) -> (160, 140)
  line L18 (160, 140) -> (50, 140)
  line L19 (50, 140) -> (50, 246.5)
  line L20 (50, 246.5) -> (-50, 246.5)
  line L21 (-50, 246.5) -> (-50, 60)
  line L22 (50, 120) -> (160, 120)
  line L23 (160, 120) -> (160, 0)
  line L24 (160, 0) -> (50, 0)
  line L25 (50, 0) -> (50, 120)
  line L26 (100, 120) -> (160, 120)
  line L27 (160, 120) -> (160, 140)
  line L28 (160, 140) -> (100, 140)
  line L29 (100, 140) -> (100, 120)
  line L30 (80, 140) -> (100, 140)
  line L31 (100, 140) -> (100, 160)
  line L32 (100, 160) -> (80, 160)
  line L33 (80, 160) -> (80, 140)
  constraint horizontal L22
  constraint vertical L23
  constraint horizontal L24
  constraint vertical L25
  constraint coincident L16.end L17.start
  constraint horizontal L26
  constraint vertical L27
  constraint horizontal L28
  constraint vertical L29
  constraint coincident L17.end L18.start
  constraint coincident L22 L26.start
  constraint horizontal L30
  constraint vertical L31
  constraint horizontal L32
  constraint vertical L33
  constraint coincident L18 L30.start
extrude "Extrude38" add sketch "Sketch48" along normal blind 30 contours L16 L17 L22 L23 L24 L25 L26 | L17 L18 L22 L26 L27 L28 L29
sketch "Sketch49" plane through (-50, 0, 0) normal (1, 0, 0) x (0, 1, 0)
  line L0 (50, 120) -> (50, 0)
  line L1 (50, 0) -> (80, 0)
  line L2 (80, 0) -> (80, 120)
  line L3 (80, 120) -> (50, 120)
  line L4 (50, 120) -> (80, 114.8826)
  line L5 (50, 114.9537) -> (50, 120)
  constraint coincident L0.start L3.end
  constraint coincident L2 L4.end
  constraint coincident L0 L5.start
extrude "Extrude39" cut sketch "Sketch49" against normal blind 50 contours L2 L3 L4
sketch "Sketch50" plane through (-50, 0, 0) normal (1, 0, 0) x (0, 1, 0)
  line L0 (80, 114.8826) -> (50, 120)
  line L1 (50, 120) -> (50, 0)
  line L2 (50, 0) -> (80, 0)
  line L3 (80, 0) -> (80, 114.8826)
  line L4 (50, 120) -> (80, 110)
  line L5 (80, 120) -> (80, 110)
  constraint coincident L0.end L1.start
  constraint coincident L3 L4.end
  constraint parallel L3 L5
extrude "Extrude40" cut sketch "Sketch50" against normal blind 50 contours L0 L3 L4 L5
sketch "Sketch51" plane through (-100, 0, 0) normal (1, 0, 0) x (0, 1, 0)
  line L0 (50, 140) -> (50, 120)
  line L1 (50, 120) -> (80, 110)
  line L2 (80, 110) -> (80, 140)
  line L3 (80, 140) -> (50, 140)
  line L4 (50, 140) -> (82, 129)
  line L5 (82, 129) -> (82, 142)
  line L6 (82, 142) -> (50, 140)
  constraint coincident L0.start L3.end
  constraint perpendicular L3 L5
extrude "Extrude41" cut sketch "Sketch51" against normal blind 65 contours L2 L3 L4
sketch "Sketch52" plane through (0, 50, 0) normal (0, 1, 0) x (-1, 0, 0)
  line L0 (100, 120) -> (100, 140)
  line L1 (100, 140) -> (50, 140)
  line L2 (50, 140) -> (50, 246.5)
  line L3 (50, 246.5) -> (-50, 246.5)
  line L4 (-50, 246.5) -> (-50, 60)
  line L5 (-50, 60) -> (7.3284, 60)
  line L6 (7.3284, 60) -> (7.3284, 50)
  line L7 (7.3284, 50) -> (-50, 50)
  line L8 (-50, 50) -> (-50, 0)
  line L9 (-50, 0) -> (50, 0)
  line L10 (50, 0) -> (50, 120)
  line L11 (50, 120) -> (100, 120)
  line L12 (-30, 63.25) -> (-30, 113.25)
  line L13 (-30, 113.25) -> (30, 113.25)
  line L14 (30, 113.25) -> (30, 63.25)
  line L15 (30, 63.25) -> (-30, 63.25)
  line L16 (20, 218.25) -> (20, 153.25)
  line L17 (20, 153.25) -> (5, 153.25)
  line L18 (5, 153.25) -> (5, 218.25)
  line L19 (5, 218.25) -> (20, 218.25)
  line L20 (-20, 218.25) -> (-5, 218.25)
  line L21 (-5, 218.25) -> (-5, 153.25)
  line L22 (-5, 153.25) -> (-20, 153.25)
  line L23 (-20, 153.25) -> (-20, 218.25)
  line L24 (100, 140) -> (80, 140)
  line L25 (80, 140) -> (80, 160)
  line L26 (80, 160) -> (100, 160)
  line L27 (100, 160) -> (100, 140)
  constraint horizontal L24
  constraint vertical L25
  constraint horizontal L26
  constraint vertical L27
  constraint coincident L0.end L1.start
extrude "Extrude42" add sketch "Sketch52" against normal blind 20 contours L1 L24 L25 L26 L27
sketch "Sketch53" plane through (0, 80, 0) normal (0, 1, 0) x (-1, 0, 0)
  line L0 (160, 129.6875) -> (100, 129.6875)
  line L1 (100, 129.6875) -> (100, 110)
  line L2 (100, 110) -> (50, 110)
  line L3 (50, 110) -> (50, 0)
  line L4 (50, 0) -> (160, 0)
  line L5 (160, 0) -> (160, 129.6875)
  line L6 (60, 100) -> (90, 100)
  line L7 (90, 100) -> (90, 70)
  line L8 (90, 70) -> (60, 70)
  line L9 (60, 70) -> (60, 100)
  line L10 (110, 100) -> (125.187, 100)
  line L11 (125.187, 100) -> (125.187, 119.8438)
  line L12 (125.187, 119.8438) -> (110, 119.8438)
  line L13 (110, 119.8438) -> (110, 100)
  line L14 (135.1028, 119.8438) -> (150, 119.8438)
  line L15 (150, 119.8438) -> (150, 100)
  line L16 (150, 100) -> (135.1028, 100)
  line L17 (135.1028, 100) -> (135.1028, 119.8438)
  constraint horizontal L6
  constraint vertical L7
  constraint horizontal L8
  constraint vertical L9
  constraint horizontal L10
  constraint vertical L11
  constraint horizontal L12
  constraint vertical L13
  constraint horizontal L14
  constraint vertical L15
  constraint horizontal L16
  constraint vertical L17
extrude "Extrude43" cut sketch "Sketch53" against normal blind 5 contours L6 L7 L8 L9 | L10 L11 L12 L13 | L14 L15 L16 L17
